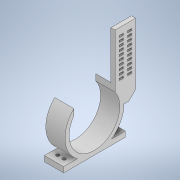
# Autodesk Inventor part: LockMount
Saved by Autodesk Inventor 2020 (Build 240168000, 168)
## iProperties
Created: 2020-06-07
Part Number: LockMount
Material: Generic
Document SubType Name: Modeling
Designer: Brandon
Density: 1 g/cm^3
Appearance: Default
Author: Brandon
Autodesk Inventor part; units mm, degrees
ref_plane "YZ Plane" through (0, 0, 0) normal (1, 0, 0) x (0, 1, 0)
ref_plane "XZ Plane" through (0, 0, 0) normal (0, 1, 0) x (-1, 0, 0)
ref_plane "XY Plane" through (0, 0, 0) normal (0, 0, 1) x (1, 0, 0)
sketch "Sketch1" plane through (0, 0, 0) normal (1, 0, 0) x (0, 1, 0)
  circle A0 centre (0, 0) radius 23.495
  circle A1 centre (0, 0) radius 27.305
  line L0 (-27.305, 28.575) -> (-22.225, 28.575)
  line L1 (-22.225, 28.575) -> (-22.225, -28.575)
  line L2 (-22.225, -28.575) -> (-27.305, -28.575)
  line L3 (-27.305, -28.575) -> (-27.305, 28.575)
  line L4 (13.7518, 19.05) -> (13.7518, -19.05)
  line L5 (13.7518, 19.05) -> (19.5617, 19.05)
  line L6 (13.7518, -19.05) -> (19.5617, -19.05)
  point P0 (-22.225, 15.8623)
  point P1 (-22.225, -15.8623)
  dimension "d0" = 46.99
  dimension "d1" = 54.61
  dimension "d2" = 5.08
  dimension "d5" = 38.1
  dimension "d11" = 57.15
  dimension "d12" = 28.575
  constraints: 14 end point, 5 point on circle, 3 parallel, 2 centre point, 2 coincident, 2 horizontal, 1 perpendicular, 1 vertical
  measures "d0" diameter of A0
  measures "d1" diameter of A1
  measures "d2" distance of L1.end L2.end
  measures "d5" distance of L4.start L4.end
  measures "d11" distance of L2.end L0.start
  measures "d12" distance from line of point (0, 0) L0
extrude "Extrusion1" add sketch "Sketch1" along normal blind 17.78 contours A0 L1 A1 L5 | L6 A1 L1 A0 | A0 L1 A1 | A1 L3 L0 L1 | L1 L2 L3 A1
sketch "Sketch2" plane through (17.78, 0, 0) normal (1, 0, 0) x (0, 0, -1)
  line L0 (19.05, 0) -> (38.1, 0)
  line L1 (38.1, 0) -> (38.1, 63.5)
  line L2 (38.1, 63.5) -> (19.05, 63.5)
  line L3 (19.05, 63.5) -> (19.05, 0)
  circle A0 centre (0, 0) radius 23.495
  circle A1 centre (0, 0) radius 27.305
  line L4 (19.05, 19.5617) -> (19.05, 13.7518) projected
  point P0 (19.05, 13.7518)
  point P1 (23.495, 0)
  dimension "d6" = 19.05
  dimension "d7" = 63.5
  dimension "d10" = 0
  constraints: 8 end point, 2 coincident, 2 parallel, 1 horizontal, 1 perpendicular, 4 other
  measures "d6" distance of L1.end L2.end
  measures "d7" distance between parallel lines of L2 L0
  measures "d10" distance between parallel lines of L3 L4
extrude "Extrusion2" add sketch "Sketch2" against normal blind 3.81 contours A0 L3 A1 L0 | A1 L3 L2 L1 L0 picked at (25.8542, 1.8052)
sketch "Sketch3" plane through (0, -27.305, -28.575) normal (0, -1, 0) x (1, 0, 0)
  circle A0 centre (11.8533, 50.8) radius 1.4986
  circle A1 centre (11.8533, 6.35) radius 1.4986
  line L0 (0, 57.15) -> (17.78, 57.15) projected
  line L1 (0, 0) -> (17.78, 0) projected
  line L2 (17.78, 57.15) -> (17.78, 0) projected
  circle A2 centre (5.9267, 6.35) radius 1.4986
  circle A3 centre (5.9267, 50.8) radius 1.4986
  line L3 (0, 57.15) -> (0, 0) projected
  point P0 (0, 28.575)
  dimension "d13" = 2.9972
  dimension "d14" = 2.9972
  dimension "d15" = 0
  dimension "d16" = 6.35
  dimension "d17" = 6.35
  dimension "d18" = 5.9267
  dimension "d32" = 2.9972
  dimension "d33" = 2.9972
  dimension "d34" = 5.9267
  dimension "d35" = 44.45
  dimension "d36" = 5.9267
  constraints: 4 centre point
  measures "d13" diameter of A0
  measures "d14" diameter of A1
  measures "d15" horizontal distance of A0.centre A1.centre
  measures "d16" distance from line of L0 A0.centre
  measures "d17" distance from line of L1 A1.centre
  measures "d18" distance from line of L2 A0.centre
  measures "d32" diameter of A2
  measures "d33" diameter of A3
  measures "d34" distance from line of L3 A2.centre
  measures "d35" distance of A2.centre A3.centre
  measures "d36" distance from line of L3 A3.centre
extrude "Extrusion3" cut sketch "Sketch3" against normal blind 6.35 contours A0 | A1 | A2 | A3
sketch "Sketch4" plane through (13.97, 0, 0) normal (-1, 0, 0) x (0, 0, 1)
  line L0 (-30.48, 57.15) -> (-26.67, 57.15)
  line L1 (-26.67, 57.15) -> (-26.67, 0)
  line L2 (-26.67, 0) -> (-30.48, 0)
  line L3 (-30.48, 0) -> (-30.48, 57.15)
  line L4 (-38.1, 63.5) -> (-38.1, 0) projected
  line L5 (-19.05, 63.5) -> (-38.1, 63.5) projected
  line L6 (-38.1, 0) -> (-27.305, 0) projected
  point P0 (0, 0)
  dimension "d21" = 3.81
  dimension "d22" = 7.62
  dimension "d23" = 6.35
  dimension "d24" = 0
  constraints: 8 end point, 2 parallel, 1 horizontal, 1 perpendicular
  measures "d21" distance of L0.start L0.end
  measures "d22" distance between parallel lines of L4 L3
  measures "d23" distance between parallel lines of L5 L0
  measures "d24" distance between parallel lines of L6 L2
extrude "Extrusion4" add sketch "Sketch4" along normal blind 6.35
sketch "Sketch5" plane through (13.97, 0, -30.48) normal (0, 0, -1) x (-1, 0, 0)
  line L0 (0, 63.5) -> (0, 0) projected
  line L1 (0, 57.2597) -> (6.35, 9.3274)
  line L2 (6.35, 57.15) -> (6.35, 0) projected
  line L3 (-3.81, 0) -> (0, 0) projected
  line L4 (0, 0) -> (6.35, 0)
  line L5 (6.35, 0) -> (6.35, 57.15)
  line L6 (6.35, 57.15) -> (0, 57.15)
  line L7 (0, 57.15) -> (0, 0)
  point P0 (13.97, 0)
  point P1 (0.0145, 57.15)
  constraints: 10 end point, 2 parallel, 2 point on line, 1 horizontal, 1 perpendicular
extrude "Extrusion5" cut sketch "Sketch5" against normal blind 3.81 contours L6 L2 L1
chamfer "Chamfer1" distance 6.35 angle 45 1 edges at (15.875, 0, -38.1)
sketch "Sketch6" plane through (17.78, 0, 0) normal (1, 0, 0) x (0, 0, -1)
  line L0 (22.86, 57.15) -> (26.67, 57.15)
  line L1 (26.67, 57.15) -> (26.67, 55.499)
  line L2 (26.67, 55.499) -> (22.86, 55.499)
  line L3 (22.86, 55.499) -> (22.86, 57.15)
  line L4 (30.48, 57.15) -> (34.29, 57.15)
  line L5 (34.29, 57.15) -> (34.29, 55.499)
  line L6 (34.29, 55.499) -> (30.48, 55.499)
  line L7 (30.48, 55.499) -> (30.48, 57.15)
  line L8 (38.1, 63.5) -> (19.05, 63.5) projected
  line L9 (19.05, 63.5) -> (19.05, 13.7518) projected
  line L10 (38.1, 6.35) -> (38.1, 63.5) projected
  point P0 (0, 0)
  dimension "d37" = 1.651
  dimension "d38" = 6.35
  dimension "d39" = 3.81
  dimension "d40" = 3.81
  dimension "d41" = 3.81
  dimension "d42" = 3.81
  dimension "d43" = 3.81
  constraints: 16 end point, 4 parallel, 2 horizontal, 2 perpendicular, 2 point on line
  measures "d37" distance between parallel lines of L2 L0
  measures "d38" distance between parallel lines of L4 L8
  measures "d39" distance between parallel lines of L9 L3
  measures "d40" distance from line of L4.start L1
  measures "d41" distance of L0.start L0.end
  measures "d42" distance of L4.start L4.end
  measures "d43" distance between parallel lines of L10 L5
extrude "Extrusion6" cut sketch "Sketch6" against normal blind 6.35
pattern_linear "Rectangular Pattern1" count 10 spacing 3.81 along (0, -1, 0) of "Extrusion6"
body "Solid1"
